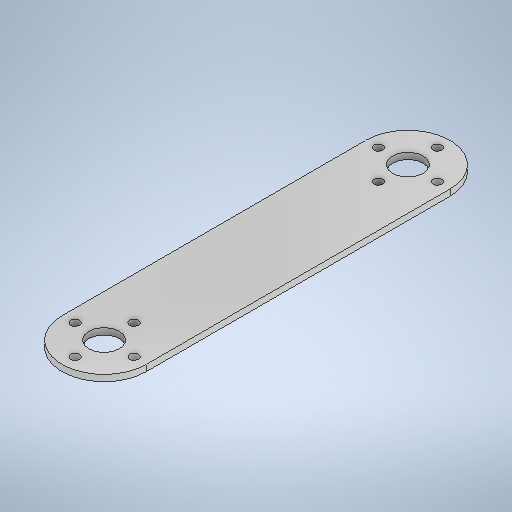
# Autodesk Inventor part: axis_10_11-connector_frame
Saved by Autodesk Inventor 2025.2 (Build 292293000, 293)
## iProperties
Created: 2025-05-04
Part Number: axis_10_11-connector_frame
Material: Aluminum 6061-AHC
Document SubType Name: Sheet Metal
Designer: User
Density: 2.7 g/cm^3
Sheet Metal Rule: Default_mm
Appearance: Aluminum - Dark
Flat Pattern Width: 2 cm
Flat Pattern Length: 9.21 cm
Flat Pattern Area: 18.42 cm^2
Sheet Metal Width: 20.000 mm
Sheet Metal Length: 92.100 mm
Sheet Metal Area: 1842.000 mm^2
Author: User
Autodesk Inventor part; units mm, degrees
ref_plane "YZ Plane" through (0, 0, 0) normal (1, 0, 0) x (0, 1, 0)
ref_plane "XZ Plane" through (0, 0, 0) normal (0, 1, 0) x (-1, 0, 0)
ref_plane "XY Plane" through (0, 0, 0) normal (0, 0, 1) x (1, 0, 0)
sketch "Sketch1" plane through (0, 0, 0) normal (0, 1, 0) x (-1, 0, 0)
  line L0 (10, -45) -> (-10, -45)
  line L1 (-10, -45) -> (-10, 47.1)
  line L2 (-10, 47.1) -> (10, 47.1)
  line L3 (10, 47.1) -> (10, -45)
  point P0 (0, 0)
  dimension "d0" = 20
  dimension "d1" = 92.1
  dimension "d2" = 45
  dimension "d3" = 10
  measures "d0" distance of L0.start L0.end
  measures "d1" distance of L0.end L1.end
  measures "d2" distance from line of L0 point (0, 0)
  measures "d3" distance from line of point (0, 0) L1
extrude "Plate1" add sketch "Sketch1" along normal blind 1.5
sketch "Sketch2" plane through (0, 0, 0) normal (0, -1, 0) x (1, 0, 0)
  circle A0 centre (0, 42) radius 0.7835 projected
  circle A1 centre (-7, 35) radius 0.7835 projected
  circle A2 centre (0, 28) radius 0.7835 projected
  circle A3 centre (7, 35) radius 0.7835 projected
  circle A4 centre (0, -28) radius 0.7835 projected
  circle A5 centre (-7, -35) radius 0.7835 projected
  circle A6 centre (0, -42) radius 0.7835 projected
  circle A7 centre (7, -35) radius 0.7835 projected
  circle A8 centre (-7, 37) radius 0.7835
  circle A9 centre (0, 30) radius 0.7835
  circle A10 centre (0, 44) radius 0.7835
  circle A11 centre (7, 37) radius 0.7835
  point P0 (0, 0)
  constraints: 4 centre point, 8 other
hole "Hole1" at (-7, 0, -35) at (7, 0, -35) at (0, 0, -42) at (0, 0, -28) at (7, 0, 37) at (0, 0, 44) at (-7, 0, 37) at (0, 0, 30) direction (0, 1, 0) diameter 2.1 depth 1.5
sketch "Sketch3" plane through (0, 1.5, 0) normal (0, 1, 0) x (1, 0, 0)
  arc A0 (10, 35) -> (-10, 35) centre (0, 35) ccw
  arc A1 (-10, -37.1) -> (10, -37.1) centre (0, -37.1) ccw
  line L0 (-10, 35) -> (-10, -37.1)
  line L1 (10, 35) -> (10, -37.1)
  line L2 (10, 45) -> (10, -47.1) projected
  line L3 (-10, 45) -> (10, 45)
  line L4 (10, 45) -> (10, -47.1)
  line L5 (10, -47.1) -> (-10, -47.1)
  line L6 (-10, -47.1) -> (-10, 45)
  point P0 (0, 0)
  point P1 (0, 45)
  point P2 (10, 45)
  point P3 (10, 35)
  point P4 (-10, -37.1)
  point P5 (0, -47.1)
  point P6 (10, -37.1)
  point P7 (1.4107, 44.9)
  point P8 (10, 35)
  point P9 (10, -37.1)
  dimension "d12" = 35
  dimension "d13" = 37.1
  dimension "d14" = 10
  dimension "d15" = 10
  dimension "d16" = 10
  dimension "d17" = 20
  dimension "d18" = 92.1
  constraints: 12 end point, 4 point on circle, 4 tangent, 3 parallel, 2 centre point, 1 horizontal, 1 perpendicular
  measures "d12" distance of point (0, 0) A0.centre
  measures "d13" distance of point (0, 0) A1.centre
  measures "d14" radius of A0
  measures "d15" radius of A1
  measures "d16" distance from line of point (0, 0) L1
  measures "d17" distance of L3.start L3.end
  measures "d18" distance of L5.end L3.start
extrude "Extrusion1" cut sketch "Sketch3" against normal blind 10 contours A0 L3 L2 | A0 L6 L3 | L2 L5 A1 | L5 L6 A1
sketch "Sketch4" plane through (0, 0, 0) normal (0, -1, 0) x (1, 0, 0)
  arc A0 (-10, -35) -> (10, -35) centre (0, -35) ccw projected
  arc A1 (10, 37.1) -> (-10, 37.1) centre (0, 37.1) ccw projected
  point P0 (0, 0)
hole "Hole2" at (0, 0, 37.1) at (0, 0, -35) direction (0, 1, 0) diameter 7.2 depth 1.5
equation "\"d10\" = Thickness"
equation "\"d26\" = Thickness"
equation "\"d4\" = Thickness"
equation "\"BendReliefWidth\" = Thickness"
equation "\"BendReliefDepth\" = 0.5 * Thickness"
equation "\"CornerReliefSize\" = 4 * Thickness"
equation "\"MinimumRemnant\" = 2 * Thickness"
equation "\"TransitionRadius\" = BendRadius"
equation "\"JacobiRadiusSize\" = BendRadius"
equation "\"GapSize\" = Thickness"
equation "\"Thickness\" = 1.5"
equation "\"BendRadius\" = 0.31"
body "Solid1"
